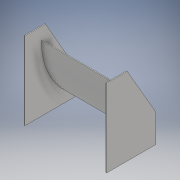
# Autodesk Inventor part: R-wing
Saved by Autodesk Inventor 2018.1 (Build 221171000, 171)
## iProperties
Created: 2017-10-11
Part Number: R-wing
Material: 一般
Document SubType Name: Modeling
Designer: kuwano
Density: 1 g/cm^3
Appearance: 既定
Author: kuwano
Autodesk Inventor part; units mm, degrees
ref_plane "YZ Plane" through (0, 0, 0) normal (1, 0, 0) x (0, 1, 0)
ref_plane "XZ Plane" through (0, 0, 0) normal (0, 1, 0) x (-1, 0, 0)
ref_plane "XY Plane" through (0, 0, 0) normal (0, 0, 1) x (1, 0, 0)
sketch "スケッチ1" plane through (0, 0, 0) normal (1, 0, 0) x (0, 1, 0)
  line L0 (10, 300) -> (0, 300)
  arc A0 (0, 300) -> (269.2388, -350) centre (919.2388, 300) ccw
  line L1 (0, -512.133) -> (0, 435.3555) projected
  arc A1 (10, 300) -> (276.3099, -342.9289) centre (919.2388, 300) ccw
  line L2 (-261.4236, 0) -> (1116.0159, 0) projected
  line L3 (276.3099, -342.9289) -> (269.2388, -350)
  point P0 (0, 0)
  dimension "d0" = 300
  dimension "d1" = 10
  dimension "d2" = 45
  dimension "d3" = 350
  constraints: 4 end point, 4 point on circle, 2 centre point, 2 line through centre, 1 concentric, 1 horizontal, 1 tangent
  measures "d0" distance between parallel lines of L2 L0
  measures "d1" distance of L0.start L0.end
  measures "d2" angle of L3 L0
  measures "d3" distance from line of L2 L3.end
extrude "押し出し1" add sketch "スケッチ1" along normal mid plane 990 contours A1 L2 A0 L0 | A1 L3 A0 L2
sketch "スケッチ2" plane through (495, 0, 0) normal (1, 0, 0) x (0, 0, -1)
  line L0 (-450, 50) -> (-450, -200)
  line L1 (-450, -200) -> (500, -200)
  line L2 (500, -200) -> (500, 400)
  line L3 (500, 400) -> (156.2178, 400)
  line L4 (156.2178, 400) -> (-450, 50)
  line L5 (690, 0) -> (-640, 0) projected
  line L6 (-300, 10) -> (-300, 0) projected
  point P0 (0, 0)
  point P1 (350, 269.2388)
  dimension "d6" = 200
  dimension "d7" = 150
  dimension "d8" = 600
  dimension "d9" = 150
  dimension "d10" = 30
  dimension "d11" = 250
  constraints: 10 end point, 3 perpendicular, 1 vertical
  measures "d6" distance between parallel lines of L1 L5
  measures "d7" distance between parallel lines of L0 L6
  measures "d8" distance of L1.end L2.end
  measures "d9" distance from line of L2 point (350, 269.239)
  measures "d10" angle of L5 L4
  measures "d11" distance of L0.start L0.end
extrude "押し出し2" add sketch "スケッチ2" along normal blind 10
mirror "ミラー1" about plane through (0, 0, 0) normal (1, 0, 0) of "押し出し2"
